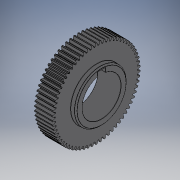
# Autodesk Inventor part: Component 16 (Sun Wheel)
Saved by Autodesk Inventor 2018 (Build 220112000, 112)
## iProperties
Created: 2023-03-15
Part Number: Component 16 (Sun Wheel)
Material: Generic
Document SubType Name: Modeling
Designer: Habib Mohamed
Density: 1 g/cm^3
Appearance: Semi-Polished
Author: Habib Mohamed
Autodesk Inventor part; units mm, degrees
(part 1 of 2)
ref_plane "YZ Plane" through (0, 0, 0) normal (1, 0, 0) x (0, 1, 0)
ref_plane "XZ Plane" through (0, 0, 0) normal (0, 1, 0) x (-1, 0, 0)
ref_plane "XY Plane" through (0, 0, 0) normal (0, 0, 1) x (1, 0, 0)
sketch "Sketch1" plane through (0, 0, 0) normal (1, 0, 0) x (0, 1, 0)
  line L0 (0, 0) -> (37.2988, 0) construction
  circle A0 centre (0, 0) radius 7.5
  line L1 (26.8131, 0.57) -> (11.4917, 0.57) construction
  line L2 (26.8131, 0.135) -> (10.3628, 0.135) construction
  arc A1 (16.9383, 0.2272) -> (15.9435, 0.5528) centre (14.4593, -5.6624) ccw
  arc A2 (16.9995, 0.135) -> (16.9383, 0.2272) centre (16.8995, 0.135) ccw
  arc A3 (15.8669, 0.646) -> (15.9435, 0.5528) centre (15.9668, 0.6501) ccw
  arc A4 (15.9435, -0.5528) -> (16.9383, -0.2272) centre (14.4593, 5.6624) ccw
  arc A5 (16.9383, -0.2272) -> (16.9995, -0.1358) centre (16.8995, -0.135) ccw
  arc A6 (15.9435, -0.5528) -> (15.8669, -0.646) centre (15.9668, -0.6501) ccw
  arc A7 (16.9097, 1.7503) -> (16.84, 1.8362) centre (16.8101, 1.7408) ccw
  arc A8 (15.7336, 2.1514) -> (15.8188, 2.0659) centre (15.8327, 2.1649) ccw
  arc A9 (16.8832, 1.3839) -> (16.9354, 1.4807) centre (16.8358, 1.472) ccw
  arc A10 (15.9239, 0.9652) -> (16.8832, 1.3839) centre (13.8556, 7.0112) ccw
  arc A11 (15.9239, 0.9652) -> (15.8564, 0.8651) centre (15.9563, 0.8706) ccw
  arc A12 (16.84, 1.8362) -> (15.8188, 2.0659) centre (14.9321, -4.2623) ccw
  arc A13 (16.6667, 3.3497) -> (16.5892, 3.4286) centre (16.5685, 3.3308) ccw
  arc A14 (15.4579, 3.6372) -> (15.5508, 3.5602) centre (15.5552, 3.6601) ccw
  arc A15 (16.6752, 2.9825) -> (16.718, 3.0838) centre (16.6196, 3.0657) ccw
  arc A16 (15.76, 2.4745) -> (16.6752, 2.9825) centre (13.1264, 8.2965) ccw
  arc A17 (15.76, 2.4745) -> (15.7024, 2.3685) centre (15.8013, 2.3834) ccw
  arc A18 (16.5892, 3.4286) -> (15.5508, 3.5602) centre (15.2696, -2.8236) ccw
  arc A19 (16.2728, 4.9188) -> (16.1881, 4.99) centre (16.1769, 4.8907) ccw
  arc A20 (15.0421, 5.0901) -> (15.142, 5.0223) centre (15.1368, 5.1221) ccw
  arc A21 (16.3161, 4.5541) -> (16.3491, 4.659) centre (16.2529, 4.6316) ccw
  arc A22 (15.4535, 3.9614) -> (16.3161, 4.5541) centre (12.2783, 9.5067) ccw
  arc A23 (15.4535, 3.9614) -> (15.4061, 3.8503) centre (15.5032, 3.8746) ccw
  arc A24 (16.1881, 4.99) -> (15.142, 5.0223) centre (15.4689, -1.3594) ccw
  arc A25 (15.7316, 6.4434) -> (15.6405, 6.5062) centre (15.6387, 6.4062) ccw
  arc A26 (14.4902, 6.4969) -> (14.596, 6.4389) centre (14.5814, 6.5378) ccw
  arc A27 (15.8094, 6.0844) -> (15.8322, 6.192) centre (15.7391, 6.1556) ccw
  arc A28 (15.0069, 5.4124) -> (15.8094, 6.0844) centre (11.3191, 10.6308) ccw
  arc A29 (15.0069, 5.4124) -> (14.9704, 5.2974) centre (15.0647, 5.3307) ccw
  arc A30 (15.6405, 6.5062) -> (14.596, 6.4389) centre (15.5281, 0.1172) ccw
  arc A31 (15.0479, 7.9096) -> (14.9512, 7.9635) centre (14.959, 7.8638) ccw
  arc A32 (13.807, 7.8448) -> (13.9179, 7.7971) centre (13.8939, 7.8942) ccw
  arc A33 (15.1594, 7.5596) -> (15.1719, 7.6689) centre (15.0827, 7.6238) ccw
  arc A34 (14.4245, 6.8144) -> (15.1594, 7.5596) centre (10.2573, 11.6586) ccw
  arc A35 (14.4245, 6.8144) -> (14.3991, 6.6964) centre (14.4897, 6.7386) ccw
  arc A36 (14.9512, 7.9635) -> (13.9179, 7.7971) centre (15.4466, 1.5927) ccw
  arc A37 (14.2279, 9.3042) -> (14.1266, 9.3486) centre (14.1437, 9.2501) ccw
  arc A38 (12.9988, 9.1218) -> (13.1137, 9.0848) centre (13.0806, 9.1792) ccw
  arc A39 (14.3722, 8.9664) -> (14.3743, 9.0764) centre (14.2897, 9.023) ccw
  arc A40 (13.7115, 8.1546) -> (14.3722, 8.9664) centre (9.1026, 12.5808) ccw
  arc A41 (13.7115, 8.1546) -> (13.6973, 8.0348) centre (13.7836, 8.0854) ccw
  arc A42 (14.1266, 9.3486) -> (13.1137, 9.0848) centre (15.2253, 3.0538) ccw
  arc A43 (13.279, 10.6145) -> (13.1739, 10.6491) centre (13.2004, 10.5527) ccw
  arc A44 (12.0728, 10.3161) -> (12.1907, 10.2902) centre (12.1489, 10.381) ccw
  arc A45 (13.4548, 10.292) -> (13.4464, 10.4016) centre (13.3673, 10.3404) ccw
  arc A46 (12.8742, 9.4211) -> (13.4548, 10.292) centre (7.8655, 13.3891) ccw
  arc A47 (12.8742, 9.4211) -> (12.8715, 9.3004) centre (12.9526, 9.359) ccw
  arc A48 (13.1739, 10.6491) -> (12.1907, 10.2902) centre (14.866, 4.4872) ccw
  arc A49 (12.2099, 11.8287) -> (12.102, 11.8531) centre (12.1376, 11.7597) ccw
  arc A50 (11.0376, 11.4169) -> (11.1574, 11.4024) centre (11.1071, 11.4888) ccw
  arc A51 (12.4156, 11.5243) -> (12.3968, 11.6327) centre (12.3239, 11.5643) ccw
  arc A52 (11.9204, 10.6022) -> (12.4156, 11.5243) centre (6.5572, 14.0761) ccw
  arc A53 (11.9204, 10.6022) -> (11.9292, 10.4818) centre (12.0043, 10.5478) ccw
  arc A54 (12.102, 11.8531) -> (11.1574, 11.4024) centre (14.3722, 5.88) ccw
  arc A55 (11.0303, 12.9357) -> (10.9205, 12.9498) centre (10.9648, 12.8602) ccw
  arc A56 (9.9023, 12.4144) -> (10.023, 12.4114) centre (9.9647, 12.4926) ccw
  arc A57 (11.2639, 12.6523) -> (11.2349, 12.7584) centre (11.1688, 12.6834) ccw
  arc A58 (10.8586, 11.6873) -> (11.2639, 12.6523) centre (5.1895, 14.6357) ccw
  arc A59 (10.8586, 11.6873) -> (10.8788, 11.5683) centre (10.9473, 11.6411) ccw
  arc A60 (10.9205, 12.9498) -> (10.023, 12.4114) centre (13.7482, 7.2195) ccw
  arc A61 (9.7507, 13.9257) -> (9.6401, 13.9293) centre (9.6927, 13.8442) ccw
  arc A62 (8.6774, 13.2995) -> (8.7978, 13.3079) centre (8.7321, 13.3832) ccw
  arc A63 (10.0102, 13.6657) -> (9.9713, 13.7686) centre (9.9126, 13.6876) ccw
  arc A64 (9.6985, 12.6665) -> (10.0102, 13.6657) centre (3.7748, 15.0627) ccw
  arc A65 (9.6985, 12.6665) -> (9.7299, 12.55) centre (9.7912, 12.629) ccw
  arc A66 (9.6401, 13.9293) -> (8.7978, 13.3079) centre (12.9997, 8.4937) ccw
  arc A67 (8.3828, 14.7895) -> (8.2724, 14.7825) centre (8.3328, 14.7029) ccw
  arc A68 (7.3739, 14.0641) -> (7.493, 14.0839) centre (7.4204, 14.1527) ccw
  arc A69 (8.6659, 14.5554) -> (8.6173, 14.6541) centre (8.5666, 14.5679) ccw
  arc A70 (8.4505, 13.5311) -> (8.6659, 14.5554) centre (2.3259, 15.3533) ccw
  arc A71 (8.4505, 13.5311) -> (8.4929, 13.4181) centre (8.5464, 13.5026) ccw
  arc A72 (8.2724, 14.7825) -> (7.493, 14.0839) centre (12.1334, 9.6909) ccw
  arc A73 (6.939, 15.5193) -> (6.8298, 15.5019) centre (6.8975, 15.4284) ccw
  arc A74 (6.0037, 14.7014) -> (6.1203, 14.7324) centre (6.0415, 14.794) ccw
  arc A75 (7.243, 15.3132) -> (7.1854, 15.4068) centre (7.1431, 15.3162) ccw
  arc A76 (7.1261, 14.2731) -> (7.243, 15.3132) centre (0.8559, 15.5049) ccw
  arc A77 (7.1261, 14.2731) -> (7.179, 14.1646) centre (7.2242, 14.2538) ccw
  arc A78 (6.8298, 15.5019) -> (6.1203, 14.7324) centre (11.1573, 10.8004) ccw
  arc A79 (5.4324, 16.1087) -> (5.3253, 16.081) centre (5.3997, 16.0142) ccw
  arc A80 (4.579, 15.2055) -> (4.6922, 15.2475) centre (4.6079, 15.3012) ccw
  arc A81 (5.7546, 15.9324) -> (5.6883, 16.0201) centre (5.6548, 15.9259) ccw
  arc A82 (5.7371, 14.8858) -> (5.7546, 15.9324) centre (-0.6218, 15.516) ccw
  arc A83 (5.7371, 14.8858) -> (5.8, 14.7829) centre (5.8366, 14.876) ccw
  arc A84 (5.3253, 16.081) -> (4.6922, 15.2475) centre (10.0801, 11.8121) ccw
  arc A85 (3.8766, 16.5521) -> (3.7726, 16.5143) centre (3.853, 16.4549) ccw
  arc A86 (3.1129, 15.5719) -> (3.2216, 15.6245) centre (3.1325, 15.67) ccw
  arc A87 (4.2141, 16.4072) -> (4.1397, 16.4883) centre (4.1154, 16.3913) ccw
  arc A88 (4.2961, 15.3638) -> (4.2141, 16.4072) centre (-2.0939, 15.3867) ccw
  arc A89 (4.2961, 15.3638) -> (4.3686, 15.2673) centre (4.3961, 15.3634) ccw
  arc A90 (3.7726, 16.5143) -> (3.2216, 15.6245) centre (8.9117, 12.7168) ccw
  arc A91 (2.2856, 16.8456) -> (2.1857, 16.7982) centre (2.2714, 16.7467) ccw
  arc A92 (1.6186, 15.7973) -> (1.7218, 15.8599) centre (1.6288, 15.8968) ccw
  arc A93 (2.6354, 16.7335) -> (2.5537, 16.8071) centre (2.5387, 16.7082) ccw
  arc A94 (2.8162, 15.7026) -> (2.6354, 16.7335) centre (-3.547, 15.118) ccw
  arc A95 (2.8162, 15.7026) -> (2.8976, 15.6134) centre (2.9158, 15.7117) ccw
  arc A96 (2.1857, 16.7982) -> (1.7218, 15.8599) centre (7.6625, 13.5063) ccw
  arc A97 (0.674, 16.9866) -> (0.579, 16.9299) centre (0.6693, 16.8867) ccw
  arc A98 (0.1097, 15.8796) -> (0.2064, 15.9518) centre (0.1104, 15.9796) ccw
  arc A99 (1.0329, 16.9083) -> (0.9445, 16.9737) centre (0.939, 16.8739) ccw
  arc A100 (1.3108, 15.8992) -> (1.0329, 16.9083) centre (-4.968, 14.7124) ccw
  arc A101 (1.3108, 15.8992) -> (1.4003, 15.8181) centre (1.4091, 15.9178) ccw
  arc A102 (0.579, 16.9299) -> (0.2064, 15.9518) centre (6.344, 14.1735) ccw
  arc A103 (-0.9437, 16.9738) -> (-1.0329, 16.9083) centre (-0.939, 16.8739) ccw
  arc A104 (-1.4003, 15.8181) -> (-1.3108, 15.8992) centre (-1.4091, 15.9178) ccw
  arc A105 (-0.579, 16.9299) -> (-0.6732, 16.9867) centre (-0.6693, 16.8867) ccw
  arc A106 (-0.2064, 15.9518) -> (-0.579, 16.9299) centre (-6.344, 14.1735) ccw
  arc A107 (-0.2064, 15.9518) -> (-0.1097, 15.8796) centre (-0.1104, 15.9796) ccw
  arc A108 (-1.0329, 16.9083) -> (-1.3108, 15.8992) centre (4.968, 14.7124) ccw
  arc A109 (-2.5529, 16.8072) -> (-2.6354, 16.7335) centre (-2.5387, 16.7082) ccw
  arc A110 (-2.8976, 15.6134) -> (-2.8162, 15.7026) centre (-2.9158, 15.7117) ccw
  arc A111 (-2.1857, 16.7982) -> (-2.2849, 16.8458) centre (-2.2714, 16.7467) ccw
  arc A112 (-1.7218, 15.8599) -> (-2.1857, 16.7982) centre (-7.6625, 13.5063) ccw
  arc A113 (-1.7218, 15.8599) -> (-1.6186, 15.7973) centre (-1.6288, 15.8968) ccw
  arc A114 (-2.6354, 16.7335) -> (-2.8162, 15.7026) centre (3.547, 15.118) ccw
  arc A115 (-4.139, 16.4884) -> (-4.2141, 16.4072) centre (-4.1154, 16.3913) ccw
  arc A116 (-4.3686, 15.2673) -> (-4.2961, 15.3638) centre (-4.3961, 15.3634) ccw
  arc A117 (-3.7726, 16.5143) -> (-3.8758, 16.5523) centre (-3.853, 16.4549) ccw
  arc A118 (-3.2216, 15.6245) -> (-3.7726, 16.5143) centre (-8.9117, 12.7168) ccw
  arc A119 (-3.2216, 15.6245) -> (-3.1129, 15.5719) centre (-3.1325, 15.67) ccw
  arc A120 (-4.2141, 16.4072) -> (-4.2961, 15.3638) centre (2.0939, 15.3867) ccw
  arc A121 (-5.6876, 16.0204) -> (-5.7546, 15.9324) centre (-5.6548, 15.9259) ccw
  arc A122 (-5.8, 14.7829) -> (-5.7371, 14.8858) centre (-5.8366, 14.876) ccw
  arc A123 (-5.3253, 16.081) -> (-5.4316, 16.1089) centre (-5.3997, 16.0142) ccw
  arc A124 (-4.6922, 15.2475) -> (-5.3253, 16.081) centre (-10.0801, 11.8121) ccw
  arc A125 (-4.6922, 15.2475) -> (-4.579, 15.2055) centre (-4.6079, 15.3012) ccw
  arc A126 (-5.7546, 15.9324) -> (-5.7371, 14.8858) centre (0.6218, 15.516) ccw
  arc A127 (-7.1846, 15.4072) -> (-7.243, 15.3132) centre (-7.1431, 15.3162) ccw
  arc A128 (-7.179, 14.1646) -> (-7.1261, 14.2731) centre (-7.2242, 14.2538) ccw
  arc A129 (-6.8298, 15.5019) -> (-6.9383, 15.5197) centre (-6.8975, 15.4284) ccw
  arc A130 (-6.1203, 14.7324) -> (-6.8298, 15.5019) centre (-11.1573, 10.8004) ccw
  arc A131 (-6.1203, 14.7324) -> (-6.0037, 14.7014) centre (-6.0415, 14.794) ccw
  arc A132 (-7.243, 15.3132) -> (-7.1261, 14.2731) centre (-0.8559, 15.5049) ccw
  arc A133 (-8.6166, 14.6545) -> (-8.6659, 14.5554) centre (-8.5666, 14.5679) ccw
  arc A134 (-8.4929, 13.4181) -> (-8.4505, 13.5311) centre (-8.5464, 13.5026) ccw
  arc A135 (-8.2724, 14.7825) -> (-8.3821, 14.7899) centre (-8.3328, 14.7029) ccw
  arc A136 (-7.493, 14.0839) -> (-8.2724, 14.7825) centre (-12.1334, 9.6909) ccw
  arc A137 (-7.493, 14.0839) -> (-7.3739, 14.0641) centre (-7.4204, 14.1527) ccw
  arc A138 (-8.6659, 14.5554) -> (-8.4505, 13.5311) centre (-2.3259, 15.3533) ccw
  arc A139 (-9.9706, 13.769) -> (-10.0102, 13.6657) centre (-9.9126, 13.6876) ccw
  arc A140 (-9.7299, 12.55) -> (-9.6985, 12.6665) centre (-9.7912, 12.629) ccw
  arc A141 (-9.6401, 13.9293) -> (-9.75, 13.9261) centre (-9.6927, 13.8442) ccw
  arc A142 (-8.7978, 13.3079) -> (-9.6401, 13.9293) centre (-12.9997, 8.4937) ccw
  arc A143 (-8.7978, 13.3079) -> (-8.6774, 13.2995) centre (-8.7321, 13.3832) ccw
  arc A144 (-10.0102, 13.6657) -> (-9.6985, 12.6665) centre (-3.7748, 15.0627) ccw
  arc A145 (-11.2343, 12.7589) -> (-11.2639, 12.6523) centre (-11.1688, 12.6834) ccw
  arc A146 (-10.8788, 11.5683) -> (-10.8586, 11.6873) centre (-10.9473, 11.6411) ccw
  arc A147 (-10.9205, 12.9498) -> (-11.0296, 12.9363) centre (-10.9648, 12.8602) ccw
  arc A148 (-10.023, 12.4114) -> (-10.9205, 12.9498) centre (-13.7482, 7.2195) ccw
  arc A149 (-10.023, 12.4114) -> (-9.9023, 12.4144) centre (-9.9647, 12.4926) ccw
  arc A150 (-11.2639, 12.6523) -> (-10.8586, 11.6873) centre (-5.1895, 14.6357) ccw
  arc A151 (-12.3962, 11.6333) -> (-12.4156, 11.5243) centre (-12.3239, 11.5643) ccw
  arc A152 (-11.9292, 10.4818) -> (-11.9204, 10.6022) centre (-12.0043, 10.5478) ccw
  arc A153 (-12.102, 11.8531) -> (-12.2094, 11.8293) centre (-12.1376, 11.7597) ccw
  arc A154 (-11.1574, 11.4024) -> (-12.102, 11.8531) centre (-14.3722, 5.88) ccw
  arc A155 (-11.1574, 11.4024) -> (-11.0376, 11.4169) centre (-11.1071, 11.4888) ccw
  arc A156 (-12.4156, 11.5243) -> (-11.9204, 10.6022) centre (-6.5572, 14.0761) ccw
  arc A157 (-13.4459, 10.4023) -> (-13.4548, 10.292) centre (-13.3673, 10.3404) ccw
  arc A158 (-12.8715, 9.3004) -> (-12.8742, 9.4211) centre (-12.9526, 9.359) ccw
  arc A159 (-13.1739, 10.6491) -> (-13.2785, 10.6151) centre (-13.2004, 10.5527) ccw
  arc A160 (-12.1907, 10.2902) -> (-13.1739, 10.6491) centre (-14.866, 4.4872) ccw
  arc A161 (-12.1907, 10.2902) -> (-12.0728, 10.3161) centre (-12.1489, 10.381) ccw
  arc A162 (-13.4548, 10.292) -> (-12.8742, 9.4211) centre (-7.8655, 13.3891) ccw
  arc A163 (-14.3738, 9.077) -> (-14.3722, 8.9664) centre (-14.2897, 9.023) ccw
  arc A164 (-13.6973, 8.0348) -> (-13.7115, 8.1546) centre (-13.7836, 8.0854) ccw
  arc A165 (-14.1266, 9.3486) -> (-14.2274, 9.3048) centre (-14.1437, 9.2501) ccw
  arc A166 (-13.1137, 9.0848) -> (-14.1266, 9.3486) centre (-15.2253, 3.0538) ccw
  arc A167 (-13.1137, 9.0848) -> (-12.9988, 9.1218) centre (-13.0806, 9.1792) ccw
  arc A168 (-14.3722, 8.9664) -> (-13.7115, 8.1546) centre (-9.1026, 12.5808) ccw
  arc A169 (-15.1716, 7.6696) -> (-15.1594, 7.5596) centre (-15.0827, 7.6238) ccw
  arc A170 (-14.3991, 6.6964) -> (-14.4245, 6.8144) centre (-14.4897, 6.7386) ccw
  arc A171 (-14.9512, 7.9635) -> (-15.0475, 7.9103) centre (-14.959, 7.8638) ccw
  arc A172 (-13.9179, 7.7971) -> (-14.9512, 7.9635) centre (-15.4466, 1.5927) ccw
  arc A173 (-13.9179, 7.7971) -> (-13.807, 7.8448) centre (-13.8939, 7.8942) ccw
  arc A174 (-15.1594, 7.5596) -> (-14.4245, 6.8144) centre (-10.2573, 11.6586) ccw
  arc A175 (-15.8319, 6.1927) -> (-15.8094, 6.0844) centre (-15.7391, 6.1556) ccw
  arc A176 (-14.9704, 5.2974) -> (-15.0069, 5.4124) centre (-15.0647, 5.3307) ccw
  arc A177 (-15.6405, 6.5062) -> (-15.7313, 6.4441) centre (-15.6387, 6.4062) ccw
  arc A178 (-14.596, 6.4389) -> (-15.6405, 6.5062) centre (-15.5281, 0.1172) ccw
  arc A179 (-14.596, 6.4389) -> (-14.4902, 6.4969) centre (-14.5814, 6.5378) ccw
  arc A180 (-15.8094, 6.0844) -> (-15.0069, 5.4124) centre (-11.3191, 10.6308) ccw
  arc A181 (-16.3489, 4.6598) -> (-16.3161, 4.5541) centre (-16.2529, 4.6316) ccw
  arc A182 (-15.4061, 3.8503) -> (-15.4535, 3.9614) centre (-15.5032, 3.8746) ccw
  arc A183 (-16.1881, 4.99) -> (-16.2726, 4.9196) centre (-16.1769, 4.8907) ccw
  arc A184 (-15.142, 5.0223) -> (-16.1881, 4.99) centre (-15.4689, -1.3594) ccw
  arc A185 (-15.142, 5.0223) -> (-15.0421, 5.0901) centre (-15.1368, 5.1221) ccw
  arc A186 (-16.3161, 4.5541) -> (-15.4535, 3.9614) centre (-12.2783, 9.5067) ccw
  arc A187 (-16.7178, 3.0846) -> (-16.6752, 2.9825) centre (-16.6196, 3.0657) ccw
  arc A188 (-15.7024, 2.3685) -> (-15.76, 2.4745) centre (-15.8013, 2.3834) ccw
  arc A189 (-16.5892, 3.4286) -> (-16.6666, 3.3505) centre (-16.5685, 3.3308) ccw
  arc A190 (-15.5508, 3.5602) -> (-16.5892, 3.4286) centre (-15.2696, -2.8236) ccw
  arc A191 (-15.5508, 3.5602) -> (-15.4579, 3.6372) centre (-15.5552, 3.6601) ccw
  arc A192 (-16.6752, 2.9825) -> (-15.76, 2.4745) centre (-13.1264, 8.2965) ccw
  arc A193 (-16.9353, 1.4815) -> (-16.8832, 1.3839) centre (-16.8358, 1.472) ccw
  arc A194 (-15.8564, 0.8651) -> (-15.9239, 0.9652) centre (-15.9563, 0.8706) ccw
  arc A195 (-16.84, 1.8362) -> (-16.9096, 1.7511) centre (-16.8101, 1.7408) ccw
  arc A196 (-15.8188, 2.0659) -> (-16.84, 1.8362) centre (-14.9321, -4.2623) ccw
  arc A197 (-15.8188, 2.0659) -> (-15.7336, 2.1514) centre (-15.8327, 2.1649) ccw
  arc A198 (-16.8832, 1.3839) -> (-15.9239, 0.9652) centre (-13.8556, 7.0112) ccw
  arc A199 (-16.9995, -0.135) -> (-16.9383, -0.2272) centre (-16.8995, -0.135) ccw
  arc A200 (-15.8669, -0.646) -> (-15.9435, -0.5528) centre (-15.9668, -0.6501) ccw
  arc A201 (-16.9383, 0.2272) -> (-16.9995, 0.1358) centre (-16.8995, 0.135) ccw
  arc A202 (-15.9435, 0.5528) -> (-16.9383, 0.2272) centre (-14.4593, -5.6624) ccw
  arc A203 (-15.9435, 0.5528) -> (-15.8669, 0.646) centre (-15.9668, 0.6501) ccw
  arc A204 (-16.9383, -0.2272) -> (-15.9435, -0.5528) centre (-14.4593, 5.6624) ccw
  arc A205 (-16.9097, -1.7503) -> (-16.84, -1.8362) centre (-16.8101, -1.7408) ccw
  arc A206 (-15.7336, -2.1514) -> (-15.8188, -2.0659) centre (-15.8327, -2.1649) ccw
  arc A207 (-16.8832, -1.3839) -> (-16.9354, -1.4807) centre (-16.8358, -1.472) ccw
  arc A208 (-15.9239, -0.9652) -> (-16.8832, -1.3839) centre (-13.8556, -7.0112) ccw
  arc A209 (-15.9239, -0.9652) -> (-15.8564, -0.8651) centre (-15.9563, -0.8706) ccw
  arc A210 (-16.84, -1.8362) -> (-15.8188, -2.0659) centre (-14.9321, 4.2623) ccw
  arc A211 (-16.6667, -3.3497) -> (-16.5892, -3.4286) centre (-16.5685, -3.3308) ccw
  arc A212 (-15.4579, -3.6372) -> (-15.5508, -3.5602) centre (-15.5552, -3.6601) ccw
  arc A213 (-16.6752, -2.9825) -> (-16.718, -3.0838) centre (-16.6196, -3.0657) ccw
  arc A214 (-15.76, -2.4745) -> (-16.6752, -2.9825) centre (-13.1264, -8.2965) ccw
  arc A215 (-15.76, -2.4745) -> (-15.7024, -2.3685) centre (-15.8013, -2.3834) ccw
  arc A216 (-16.5892, -3.4286) -> (-15.5508, -3.5602) centre (-15.2696, 2.8236) ccw
  arc A217 (-16.2728, -4.9188) -> (-16.1881, -4.99) centre (-16.1769, -4.8907) ccw
  arc A218 (-15.0421, -5.0901) -> (-15.142, -5.0223) centre (-15.1368, -5.1221) ccw
  arc A219 (-16.3161, -4.5541) -> (-16.3491, -4.659) centre (-16.2529, -4.6316) ccw
  arc A220 (-15.4535, -3.9614) -> (-16.3161, -4.5541) centre (-12.2783, -9.5067) ccw
  arc A221 (-15.4535, -3.9614) -> (-15.4061, -3.8503) centre (-15.5032, -3.8746) ccw
  arc A222 (-16.1881, -4.99) -> (-15.142, -5.0223) centre (-15.4689, 1.3594) ccw
  arc A223 (-15.7316, -6.4434) -> (-15.6405, -6.5062) centre (-15.6387, -6.4062) ccw
  arc A224 (-14.4902, -6.4969) -> (-14.596, -6.4389) centre (-14.5814, -6.5378) ccw
  arc A225 (-15.8094, -6.0844) -> (-15.8322, -6.192) centre (-15.7391, -6.1556) ccw
  arc A226 (-15.0069, -5.4124) -> (-15.8094, -6.0844) centre (-11.3191, -10.6308) ccw
  arc A227 (-15.0069, -5.4124) -> (-14.9704, -5.2974) centre (-15.0647, -5.3307) ccw
  arc A228 (-15.6405, -6.5062) -> (-14.596, -6.4389) centre (-15.5281, -0.1172) ccw
  arc A229 (-15.0479, -7.9096) -> (-14.9512, -7.9635) centre (-14.959, -7.8638) ccw
  arc A230 (-13.807, -7.8448) -> (-13.9179, -7.7971) centre (-13.8939, -7.8942) ccw
  arc A231 (-15.1594, -7.5596) -> (-15.1719, -7.6689) centre (-15.0827, -7.6238) ccw
  arc A232 (-14.4245, -6.8144) -> (-15.1594, -7.5596) centre (-10.2573, -11.6586) ccw
  arc A233 (-14.4245, -6.8144) -> (-14.3991, -6.6964) centre (-14.4897, -6.7386) ccw
  arc A234 (-14.9512, -7.9635) -> (-13.9179, -7.7971) centre (-15.4466, -1.5927) ccw
  arc A235 (-14.2279, -9.3042) -> (-14.1266, -9.3486) centre (-14.1437, -9.2501) ccw
  arc A236 (-12.9988, -9.1218) -> (-13.1137, -9.0848) centre (-13.0806, -9.1792) ccw
  arc A237 (-14.3722, -8.9664) -> (-14.3743, -9.0764) centre (-14.2897, -9.023) ccw
  arc A238 (-13.7115, -8.1546) -> (-14.3722, -8.9664) centre (-9.1026, -12.5808) ccw
  arc A239 (-13.7115, -8.1546) -> (-13.6973, -8.0348) centre (-13.7836, -8.0854) ccw
  arc A240 (-14.1266, -9.3486) -> (-13.1137, -9.0848) centre (-15.2253, -3.0538) ccw
  arc A241 (-13.279, -10.6145) -> (-13.1739, -10.6491) centre (-13.2004, -10.5527) ccw
  arc A242 (-12.0728, -10.3161) -> (-12.1907, -10.2902) centre (-12.1489, -10.381) ccw
  arc A243 (-13.4548, -10.292) -> (-13.4464, -10.4016) centre (-13.3673, -10.3404) ccw
  arc A244 (-12.8742, -9.4211) -> (-13.4548, -10.292) centre (-7.8655, -13.3891) ccw
  arc A245 (-12.8742, -9.4211) -> (-12.8715, -9.3004) centre (-12.9526, -9.359) ccw
  arc A246 (-13.1739, -10.6491) -> (-12.1907, -10.2902) centre (-14.866, -4.4872) ccw
  arc A247 (-12.2099, -11.8287) -> (-12.102, -11.8531) centre (-12.1376, -11.7597) ccw
  arc A248 (-11.0376, -11.4169) -> (-11.1574, -11.4024) centre (-11.1071, -11.4888) ccw
  arc A249 (-12.4156, -11.5243) -> (-12.3968, -11.6327) centre (-12.3239, -11.5643) ccw
  arc A250 (-11.9204, -10.6022) -> (-12.4156, -11.5243) centre (-6.5572, -14.0761) ccw
  arc A251 (-11.9204, -10.6022) -> (-11.9292, -10.4818) centre (-12.0043, -10.5478) ccw
  arc A252 (-12.102, -11.8531) -> (-11.1574, -11.4024) centre (-14.3722, -5.88) ccw
  arc A253 (-11.0303, -12.9357) -> (-10.9205, -12.9498) centre (-10.9648, -12.8602) ccw
  arc A254 (-9.9023, -12.4144) -> (-10.023, -12.4114) centre (-9.9647, -12.4926) ccw
  arc A255 (-11.2639, -12.6523) -> (-11.2349, -12.7584) centre (-11.1688, -12.6834) ccw
  arc A256 (-10.8586, -11.6873) -> (-11.2639, -12.6523) centre (-5.1895, -14.6357) ccw
  arc A257 (-10.8586, -11.6873) -> (-10.8788, -11.5683) centre (-10.9473, -11.6411) ccw
  arc A258 (-10.9205, -12.9498) -> (-10.023, -12.4114) centre (-13.7482, -7.2195) ccw
  arc A259 (-9.7507, -13.9257) -> (-9.6401, -13.9293) centre (-9.6927, -13.8442) ccw
  arc A260 (-8.6774, -13.2995) -> (-8.7978, -13.3079) centre (-8.7321, -13.3832) ccw
  arc A261 (-10.0102, -13.6657) -> (-9.9713, -13.7686) centre (-9.9126, -13.6876) ccw
  arc A262 (-9.6985, -12.6665) -> (-10.0102, -13.6657) centre (-3.7748, -15.0627) ccw
  arc A263 (-9.6985, -12.6665) -> (-9.7299, -12.55) centre (-9.7912, -12.629) ccw
  arc A264 (-9.6401, -13.9293) -> (-8.7978, -13.3079) centre (-12.9997, -8.4937) ccw
  arc A265 (-8.3828, -14.7895) -> (-8.2724, -14.7825) centre (-8.3328, -14.7029) ccw
  arc A266 (-7.3739, -14.0641) -> (-7.493, -14.0839) centre (-7.4204, -14.1527) ccw
  arc A267 (-8.6659, -14.5554) -> (-8.6173, -14.6541) centre (-8.5666, -14.5679) ccw
  arc A268 (-8.4505, -13.5311) -> (-8.6659, -14.5554) centre (-2.3259, -15.3533) ccw
  arc A269 (-8.4505, -13.5311) -> (-8.4929, -13.4181) centre (-8.5464, -13.5026) ccw
  arc A270 (-8.2724, -14.7825) -> (-7.493, -14.0839) centre (-12.1334, -9.6909) ccw
  arc A271 (-6.939, -15.5193) -> (-6.8298, -15.5019) centre (-6.8975, -15.4284) ccw
  arc A272 (-6.0037, -14.7014) -> (-6.1203, -14.7324) centre (-6.0415, -14.794) ccw
  arc A273 (-7.243, -15.3132) -> (-7.1854, -15.4068) centre (-7.1431, -15.3162) ccw
  arc A274 (-7.1261, -14.2731) -> (-7.243, -15.3132) centre (-0.8559, -15.5049) ccw
  arc A275 (-7.1261, -14.2731) -> (-7.179, -14.1646) centre (-7.2242, -14.2538) ccw
  arc A276 (-6.8298, -15.5019) -> (-6.1203, -14.7324) centre (-11.1573, -10.8004) ccw
  arc A277 (-5.4324, -16.1087) -> (-5.3253, -16.081) centre (-5.3997, -16.0142) ccw
  arc A278 (-4.579, -15.2055) -> (-4.6922, -15.2475) centre (-4.6079, -15.3012) ccw
  arc A279 (-5.7546, -15.9324) -> (-5.6883, -16.0201) centre (-5.6548, -15.9259) ccw
  arc A280 (-5.7371, -14.8858) -> (-5.7546, -15.9324) centre (0.6218, -15.516) ccw
  arc A281 (-5.7371, -14.8858) -> (-5.8, -14.7829) centre (-5.8366, -14.876) ccw
  arc A282 (-5.3253, -16.081) -> (-4.6922, -15.2475) centre (-10.0801, -11.8121) ccw
  arc A283 (-3.8766, -16.5521) -> (-3.7726, -16.5143) centre (-3.853, -16.4549) ccw
  arc A284 (-3.1129, -15.5719) -> (-3.2216, -15.6245) centre (-3.1325, -15.67) ccw
  arc A285 (-4.2141, -16.4072) -> (-4.1397, -16.4883) centre (-4.1154, -16.3913) ccw
  arc A286 (-4.2961, -15.3638) -> (-4.2141, -16.4072) centre (2.0939, -15.3867) ccw
  arc A287 (-4.2961, -15.3638) -> (-4.3686, -15.2673) centre (-4.3961, -15.3634) ccw
  arc A288 (-3.7726, -16.5143) -> (-3.2216, -15.6245) centre (-8.9117, -12.7168) ccw
  arc A289 (-2.2856, -16.8456) -> (-2.1857, -16.7982) centre (-2.2714, -16.7467) ccw
  arc A290 (-1.6186, -15.7973) -> (-1.7218, -15.8599) centre (-1.6288, -15.8968) ccw
  arc A291 (-2.6354, -16.7335) -> (-2.5537, -16.8071) centre (-2.5387, -16.7082) ccw
  arc A292 (-2.8162, -15.7026) -> (-2.6354, -16.7335) centre (3.547, -15.118) ccw
  arc A293 (-2.8162, -15.7026) -> (-2.8976, -15.6134) centre (-2.9158, -15.7117) ccw
  arc A294 (-2.1857, -16.7982) -> (-1.7218, -15.8599) centre (-7.6625, -13.5063) ccw
  arc A295 (-0.674, -16.9866) -> (-0.579, -16.9299) centre (-0.6693, -16.8867) ccw
  arc A296 (-0.1097, -15.8796) -> (-0.2064, -15.9518) centre (-0.1104, -15.9796) ccw
  arc A297 (-1.0329, -16.9083) -> (-0.9445, -16.9737) centre (-0.939, -16.8739) ccw
  arc A298 (-1.3108, -15.8992) -> (-1.0329, -16.9083) centre (4.968, -14.7124) ccw
  arc A299 (-1.3108, -15.8992) -> (-1.4003, -15.8181) centre (-1.4091, -15.9178) ccw
  arc A300 (-0.579, -16.9299) -> (-0.2064, -15.9518) centre (-6.344, -14.1735) ccw
  arc A301 (0.9437, -16.9738) -> (1.0329, -16.9083) centre (0.939, -16.8739) ccw
  arc A302 (1.4003, -15.8181) -> (1.3108, -15.8992) centre (1.4091, -15.9178) ccw
  arc A303 (0.579, -16.9299) -> (0.6732, -16.9867) centre (0.6693, -16.8867) ccw
  arc A304 (0.2064, -15.9518) -> (0.579, -16.9299) centre (6.344, -14.1735) ccw
  arc A305 (0.2064, -15.9518) -> (0.1097, -15.8796) centre (0.1104, -15.9796) ccw
  arc A306 (1.0329, -16.9083) -> (1.3108, -15.8992) centre (-4.968, -14.7124) ccw
  arc A307 (2.5529, -16.8072) -> (2.6354, -16.7335) centre (2.5387, -16.7082) ccw
  arc A308 (2.8976, -15.6134) -> (2.8162, -15.7026) centre (2.9158, -15.7117) ccw
  arc A309 (2.1857, -16.7982) -> (2.2849, -16.8458) centre (2.2714, -16.7467) ccw
  arc A310 (1.7218, -15.8599) -> (2.1857, -16.7982) centre (7.6625, -13.5063) ccw
  arc A311 (1.7218, -15.8599) -> (1.6186, -15.7973) centre (1.6288, -15.8968) ccw
  arc A312 (2.6354, -16.7335) -> (2.8162, -15.7026) centre (-3.547, -15.118) ccw
  arc A313 (4.139, -16.4884) -> (4.2141, -16.4072) centre (4.1154, -16.3913) ccw
  arc A314 (4.3686, -15.2673) -> (4.2961, -15.3638) centre (4.3961, -15.3634) ccw
  arc A315 (3.7726, -16.5143) -> (3.8758, -16.5523) centre (3.853, -16.4549) ccw
  arc A316 (3.2216, -15.6245) -> (3.7726, -16.5143) centre (8.9117, -12.7168) ccw
  arc A317 (3.2216, -15.6245) -> (3.1129, -15.5719) centre (3.1325, -15.67) ccw
  arc A318 (4.2141, -16.4072) -> (4.2961, -15.3638) centre (-2.0939, -15.3867) ccw
  arc A319 (5.6876, -16.0204) -> (5.7546, -15.9324) centre (5.6548, -15.9259) ccw
  arc A320 (5.8, -14.7829) -> (5.7371, -14.8858) centre (5.8366, -14.876) ccw
  arc A321 (5.3253, -16.081) -> (5.4316, -16.1089) centre (5.3997, -16.0142) ccw
  arc A322 (4.6922, -15.2475) -> (5.3253, -16.081) centre (10.0801, -11.8121) ccw
  arc A323 (4.6922, -15.2475) -> (4.579, -15.2055) centre (4.6079, -15.3012) ccw
  arc A324 (5.7546, -15.9324) -> (5.7371, -14.8858) centre (-0.6218, -15.516) ccw
  arc A325 (7.1846, -15.4072) -> (7.243, -15.3132) centre (7.1431, -15.3162) ccw
  arc A326 (7.179, -14.1646) -> (7.1261, -14.2731) centre (7.2242, -14.2538) ccw
  arc A327 (6.8298, -15.5019) -> (6.9383, -15.5197) centre (6.8975, -15.4284) ccw
  arc A328 (6.1203, -14.7324) -> (6.8298, -15.5019) centre (11.1573, -10.8004) ccw
  arc A329 (6.1203, -14.7324) -> (6.0037, -14.7014) centre (6.0415, -14.794) ccw
  arc A330 (7.243, -15.3132) -> (7.1261, -14.2731) centre (0.8559, -15.5049) ccw
  arc A331 (8.6166, -14.6545) -> (8.6659, -14.5554) centre (8.5666, -14.5679) ccw
  arc A332 (8.4929, -13.4181) -> (8.4505, -13.5311) centre (8.5464, -13.5026) ccw
  arc A333 (8.2724, -14.7825) -> (8.3821, -14.7899) centre (8.3328, -14.7029) ccw
  arc A334 (7.493, -14.0839) -> (8.2724, -14.7825) centre (12.1334, -9.6909) ccw
  arc A335 (7.493, -14.0839) -> (7.3739, -14.0641) centre (7.4204, -14.1527) ccw
  arc A336 (8.6659, -14.5554) -> (8.4505, -13.5311) centre (2.3259, -15.3533) ccw
  arc A337 (9.9706, -13.769) -> (10.0102, -13.6657) centre (9.9126, -13.6876) ccw
  arc A338 (9.7299, -12.55) -> (9.6985, -12.6665) centre (9.7912, -12.629) ccw
  arc A339 (9.6401, -13.9293) -> (9.75, -13.9261) centre (9.6927, -13.8442) ccw
  arc A340 (8.7978, -13.3079) -> (9.6401, -13.9293) centre (12.9997, -8.4937) ccw
  arc A341 (8.7978, -13.3079) -> (8.6774, -13.2995) centre (8.7321, -13.3832) ccw
  arc A342 (10.0102, -13.6657) -> (9.6985, -12.6665) centre (3.7748, -15.0627) ccw
  arc A343 (11.2343, -12.7589) -> (11.2639, -12.6523) centre (11.1688, -12.6834) ccw
  arc A344 (10.8788, -11.5683) -> (10.8586, -11.6873) centre (10.9473, -11.6411) ccw
  arc A345 (10.9205, -12.9498) -> (11.0296, -12.9363) centre (10.9648, -12.8602) ccw
  arc A346 (10.023, -12.4114) -> (10.9205, -12.9498) centre (13.7482, -7.2195) ccw
  arc A347 (10.023, -12.4114) -> (9.9023, -12.4144) centre (9.9647, -12.4926) ccw
  arc A348 (11.2639, -12.6523) -> (10.8586, -11.6873) centre (5.1895, -14.6357) ccw
  arc A349 (12.3962, -11.6333) -> (12.4156, -11.5243) centre (12.3239, -11.5643) ccw
  arc A350 (11.9292, -10.4818) -> (11.9204, -10.6022) centre (12.0043, -10.5478) ccw
  arc A351 (12.102, -11.8531) -> (12.2094, -11.8293) centre (12.1376, -11.7597) ccw
  arc A352 (11.1574, -11.4024) -> (12.102, -11.8531) centre (14.3722, -5.88) ccw
  arc A353 (11.1574, -11.4024) -> (11.0376, -11.4169) centre (11.1071, -11.4888) ccw
  arc A354 (12.4156, -11.5243) -> (11.9204, -10.6022) centre (6.5572, -14.0761) ccw
  arc A355 (13.4459, -10.4023) -> (13.4548, -10.292) centre (13.3673, -10.3404) ccw
  arc A356 (12.8715, -9.3004) -> (12.8742, -9.4211) centre (12.9526, -9.359) ccw
  arc A357 (13.1739, -10.6491) -> (13.2785, -10.6151) centre (13.2004, -10.5527) ccw
  arc A358 (12.1907, -10.2902) -> (13.1739, -10.6491) centre (14.866, -4.4872) ccw
  arc A359 (12.1907, -10.2902) -> (12.0728, -10.3161) centre (12.1489, -10.381) ccw
  arc A360 (13.4548, -10.292) -> (12.8742, -9.4211) centre (7.8655, -13.3891) ccw
  arc A361 (14.3738, -9.077) -> (14.3722, -8.9664) centre (14.2897, -9.023) ccw
  arc A362 (13.6973, -8.0348) -> (13.7115, -8.1546) centre (13.7836, -8.0854) ccw
  arc A363 (14.1266, -9.3486) -> (14.2274, -9.3048) centre (14.1437, -9.2501) ccw
  arc A364 (13.1137, -9.0848) -> (14.1266, -9.3486) centre (15.2253, -3.0538) ccw
  arc A365 (13.1137, -9.0848) -> (12.9988, -9.1218) centre (13.0806, -9.1792) ccw
  arc A366 (14.3722, -8.9664) -> (13.7115, -8.1546) centre (9.1026, -12.5808) ccw
  arc A367 (15.1716, -7.6696) -> (15.1594, -7.5596) centre (15.0827, -7.6238) ccw
  arc A368 (14.3991, -6.6964) -> (14.4245, -6.8144) centre (14.4897, -6.7386) ccw
  arc A369 (14.9512, -7.9635) -> (15.0475, -7.9103) centre (14.959, -7.8638) ccw
  arc A370 (13.9179, -7.7971) -> (14.9512, -7.9635) centre (15.4466, -1.5927) ccw
  arc A371 (13.9179, -7.7971) -> (13.807, -7.8448) centre (13.8939, -7.8942) ccw
  arc A372 (15.1594, -7.5596) -> (14.4245, -6.8144) centre (10.2573, -11.6586) ccw
  arc A373 (15.8319, -6.1927) -> (15.8094, -6.0844) centre (15.7391, -6.1556) ccw
  arc A374 (14.9704, -5.2974) -> (15.0069, -5.4124) centre (15.0647, -5.3307) ccw
  arc A375 (15.6405, -6.5062) -> (15.7313, -6.4441) centre (15.6387, -6.4062) ccw
  arc A376 (14.596, -6.4389) -> (15.6405, -6.5062) centre (15.5281, -0.1172) ccw
  arc A377 (14.596, -6.4389) -> (14.4902, -6.4969) centre (14.5814, -6.5378) ccw
  arc A378 (15.8094, -6.0844) -> (15.0069, -5.4124) centre (11.3191, -10.6308) ccw
  arc A379 (16.3489, -4.6598) -> (16.3161, -4.5541) centre (16.2529, -4.6316) ccw
  arc A380 (15.4061, -3.8503) -> (15.4535, -3.9614) centre (15.5032, -3.8746) ccw
  arc A381 (16.1881, -4.99) -> (16.2726, -4.9196) centre (16.1769, -4.8907) ccw
  arc A382 (15.142, -5.0223) -> (16.1881, -4.99) centre (15.4689, 1.3594) ccw
  arc A383 (15.142, -5.0223) -> (15.0421, -5.0901) centre (15.1368, -5.1221) ccw
  arc A384 (16.3161, -4.5541) -> (15.4535, -3.9614) centre (12.2783, -9.5067) ccw
  arc A385 (16.7178, -3.0846) -> (16.6752, -2.9825) centre (16.6196, -3.0657) ccw
  arc A386 (15.7024, -2.3685) -> (15.76, -2.4745) centre (15.8013, -2.3834) ccw
  arc A387 (16.5892, -3.4286) -> (16.6666, -3.3505) centre (16.5685, -3.3308) ccw
  arc A388 (15.5508, -3.5602) -> (16.5892, -3.4286) centre (15.2696, 2.8236) ccw
  arc A389 (15.5508, -3.5602) -> (15.4579, -3.6372) centre (15.5552, -3.6601) ccw
  arc A390 (16.6752, -2.9825) -> (15.76, -2.4745) centre (13.1264, -8.2965) ccw
  arc A391 (16.9353, -1.4815) -> (16.8832, -1.3839) centre (16.8358, -1.472) ccw
  arc A392 (15.8564, -0.8651) -> (15.9239, -0.9652) centre (15.9563, -0.8706) ccw
  arc A393 (16.84, -1.8362) -> (16.9096, -1.7511) centre (16.8101, -1.7408) ccw
  arc A394 (15.8188, -2.0659) -> (16.84, -1.8362) centre (14.9321, 4.2623) ccw
  arc A395 (15.8188, -2.0659) -> (15.7336, -2.1514) centre (15.8327, -2.1649) ccw
  arc A396 (16.8832, -1.3839) -> (15.9239, -0.9652) centre (13.8556, -7.0112) ccw
  arc A397 (15.8669, 0.646) -> (15.8564, 0.8651) centre (0, 0) ccw
  arc A398 (15.7336, 2.1514) -> (15.7024, 2.3685) centre (0, 0) ccw
  arc A399 (15.4579, 3.6372) -> (15.4061, 3.8503) centre (0, 0) ccw
  arc A400 (15.0421, 5.0901) -> (14.9704, 5.2974) centre (0, 0) ccw
  arc A401 (14.4902, 6.4969) -> (14.3991, 6.6964) centre (0, 0) ccw
  arc A402 (13.807, 7.8448) -> (13.6973, 8.0348) centre (0, 0) ccw
  arc A403 (12.9988, 9.1218) -> (12.8715, 9.3004) centre (0, 0) ccw
  arc A404 (12.0728, 10.3161) -> (11.9292, 10.4818) centre (0, 0) ccw
  arc A405 (11.0376, 11.4169) -> (10.8788, 11.5683) centre (0, 0) ccw
  arc A406 (9.9023, 12.4144) -> (9.7299, 12.55) centre (0, 0) ccw
  arc A407 (8.6774, 13.2995) -> (8.4929, 13.4181) centre (0, 0) ccw
  arc A408 (7.3739, 14.0641) -> (7.179, 14.1646) centre (0, 0) ccw
  arc A409 (6.0037, 14.7014) -> (5.8, 14.7829) centre (0, 0) ccw
  arc A410 (4.579, 15.2055) -> (4.3686, 15.2673) centre (0, 0) ccw
  arc A411 (3.1129, 15.5719) -> (2.8976, 15.6134) centre (0, 0) ccw
  arc A412 (1.6186, 15.7973) -> (1.4003, 15.8181) centre (0, 0) ccw
  arc A413 (0.1097, 15.8796) -> (-0.1097, 15.8796) centre (0, 0) ccw
  arc A414 (-1.4003, 15.8181) -> (-1.6186, 15.7973) centre (0, 0) ccw
  arc A415 (-2.8976, 15.6134) -> (-3.1129, 15.5719) centre (0, 0) ccw
  arc A416 (16.9354, 1.4807) -> (16.9096, 1.7511) centre (0, 0) ccw
  arc A417 (16.718, 3.0838) -> (16.6666, 3.3505) centre (0, 0) ccw
  arc A418 (16.3491, 4.659) -> (16.2726, 4.9196) centre (0, 0) ccw
  arc A419 (15.8322, 6.192) -> (15.7313, 6.4441) centre (0, 0) ccw
  arc A420 (15.1719, 7.6689) -> (15.0475, 7.9103) centre (0, 0) ccw
  arc A421 (14.3743, 9.0764) -> (14.2274, 9.3048) centre (0, 0) ccw
  arc A422 (13.4464, 10.4016) -> (13.2785, 10.6151) centre (0, 0) ccw
  arc A423 (12.3968, 11.6327) -> (12.2094, 11.8293) centre (0, 0) ccw
  arc A424 (11.2349, 12.7584) -> (11.0296, 12.9363) centre (0, 0) ccw
  arc A425 (9.9713, 13.7686) -> (9.75, 13.9261) centre (0, 0) ccw
  arc A426 (8.6173, 14.6541) -> (8.3821, 14.7899) centre (0, 0) ccw
  arc A427 (7.1854, 15.4068) -> (6.9383, 15.5197) centre (0, 0) ccw
  arc A428 (5.6883, 16.0201) -> (5.4316, 16.1089) centre (0, 0) ccw
  arc A429 (4.1397, 16.4883) -> (3.8758, 16.5523) centre (0, 0) ccw
  arc A430 (2.5537, 16.8071) -> (2.2849, 16.8458) centre (0, 0) ccw
  arc A431 (0.9445, 16.9737) -> (0.6732, 16.9867) centre (0, 0) ccw
  arc A432 (-0.6732, 16.9867) -> (-0.9445, 16.9737) centre (0, 0) ccw
  arc A433 (-2.2849, 16.8458) -> (-2.5537, 16.8071) centre (0, 0) ccw
  arc A434 (16.9995, -0.1358) -> (16.9995, 0.1358) centre (0, 0) ccw
  arc A435 (15.8564, -0.8651) -> (15.8669, -0.646) centre (0, 0) ccw
  arc A436 (-4.3686, 15.2673) -> (-4.579, 15.2055) centre (0, 0) ccw
  arc A437 (-5.8, 14.7829) -> (-6.0037, 14.7014) centre (0, 0) ccw
  arc A438 (-7.179, 14.1646) -> (-7.3739, 14.0641) centre (0, 0) ccw
  arc A439 (-8.4929, 13.4181) -> (-8.6774, 13.2995) centre (0, 0) ccw
  arc A440 (-9.7299, 12.55) -> (-9.9023, 12.4144) centre (0, 0) ccw
  arc A441 (-10.8788, 11.5683) -> (-11.0376, 11.4169) centre (0, 0) ccw
  arc A442 (-11.9292, 10.4818) -> (-12.0728, 10.3161) centre (0, 0) ccw
  arc A443 (-12.8715, 9.3004) -> (-12.9988, 9.1218) centre (0, 0) ccw
  arc A444 (-13.6973, 8.0348) -> (-13.807, 7.8448) centre (0, 0) ccw
  arc A445 (-14.3991, 6.6964) -> (-14.4902, 6.4969) centre (0, 0) ccw
  arc A446 (-14.9704, 5.2974) -> (-15.0421, 5.0901) centre (0, 0) ccw
  arc A447 (-15.4061, 3.8503) -> (-15.4579, 3.6372) centre (0, 0) ccw
  arc A448 (-15.7024, 2.3685) -> (-15.7336, 2.1514) centre (0, 0) ccw
  arc A449 (-15.8564, 0.8651) -> (-15.8669, 0.646) centre (0, 0) ccw
  arc A450 (-15.8669, -0.646) -> (-15.8564, -0.8651) centre (0, 0) ccw
  arc A451 (-15.7336, -2.1514) -> (-15.7024, -2.3685) centre (0, 0) ccw
  arc A452 (-15.4579, -3.6372) -> (-15.4061, -3.8503) centre (0, 0) ccw
  arc A453 (-15.0421, -5.0901) -> (-14.9704, -5.2974) centre (0, 0) ccw
  arc A454 (-14.4902, -6.4969) -> (-14.3991, -6.6964) centre (0, 0) ccw
  arc A455 (-13.807, -7.8448) -> (-13.6973, -8.0348) centre (0, 0) ccw
  arc A456 (-12.9988, -9.1218) -> (-12.8715, -9.3004) centre (0, 0) ccw
  arc A457 (-12.0728, -10.3161) -> (-11.9292, -10.4818) centre (0, 0) ccw
  arc A458 (-11.0376, -11.4169) -> (-10.8788, -11.5683) centre (0, 0) ccw
  arc A459 (-9.9023, -12.4144) -> (-9.7299, -12.55) centre (0, 0) ccw
  arc A460 (-3.8758, 16.5523) -> (-4.1397, 16.4883) centre (0, 0) ccw
  arc A461 (-5.4316, 16.1089) -> (-5.6883, 16.0201) centre (0, 0) ccw
  arc A462 (-6.9383, 15.5197) -> (-7.1854, 15.4068) centre (0, 0) ccw
  arc A463 (-8.3821, 14.7899) -> (-8.6173, 14.6541) centre (0, 0) ccw
  arc A464 (-9.75, 13.9261) -> (-9.9713, 13.7686) centre (0, 0) ccw
  arc A465 (-11.0296, 12.9363) -> (-11.2349, 12.7584) centre (0, 0) ccw
  arc A466 (-12.2094, 11.8293) -> (-12.3968, 11.6327) centre (0, 0) ccw
  arc A467 (-13.2785, 10.6151) -> (-13.4464, 10.4016) centre (0, 0) ccw
  arc A468 (-14.2274, 9.3048) -> (-14.3743, 9.0764) centre (0, 0) ccw
  arc A469 (-15.0475, 7.9103) -> (-15.1719, 7.6689) centre (0, 0) ccw
  arc A470 (-15.7313, 6.4441) -> (-15.8322, 6.192) centre (0, 0) ccw
  arc A471 (-16.2726, 4.9196) -> (-16.3491, 4.659) centre (0, 0) ccw
  arc A472 (-16.6666, 3.3505) -> (-16.718, 3.0838) centre (0, 0) ccw
  arc A473 (-16.9096, 1.7511) -> (-16.9354, 1.4807) centre (0, 0) ccw
  arc A474 (-16.9995, 0.1358) -> (-16.9995, -0.1358) centre (0, 0) ccw
  arc A475 (-16.9354, -1.4807) -> (-16.9096, -1.7511) centre (0, 0) ccw
  arc A476 (-16.718, -3.0838) -> (-16.6666, -3.3505) centre (0, 0) ccw
  arc A477 (-16.3491, -4.659) -> (-16.2726, -4.9196) centre (0, 0) ccw
  arc A478 (-15.8322, -6.192) -> (-15.7313, -6.4441) centre (0, 0) ccw
  arc A479 (-15.1719, -7.6689) -> (-15.0475, -7.9103) centre (0, 0) ccw
  arc A480 (-14.3743, -9.0764) -> (-14.2274, -9.3048) centre (0, 0) ccw
  arc A481 (-13.4464, -10.4016) -> (-13.2785, -10.6151) centre (0, 0) ccw
  arc A482 (-12.3968, -11.6327) -> (-12.2094, -11.8293) centre (0, 0) ccw
  arc A483 (-11.2349, -12.7584) -> (-11.0296, -12.9363) centre (0, 0) ccw
  arc A484 (16.9096, -1.7511) -> (16.9354, -1.4807) centre (0, 0) ccw
  arc A485 (16.6666, -3.3505) -> (16.718, -3.0838) centre (0, 0) ccw
  arc A486 (16.2726, -4.9196) -> (16.3491, -4.659) centre (0, 0) ccw
  arc A487 (15.7313, -6.4441) -> (15.8322, -6.192) centre (0, 0) ccw
  arc A488 (15.0475, -7.9103) -> (15.1719, -7.6689) centre (0, 0) ccw
  arc A489 (14.2274, -9.3048) -> (14.3743, -9.0764) centre (0, 0) ccw
  arc A490 (13.2785, -10.6151) -> (13.4464, -10.4016) centre (0, 0) ccw
  arc A491 (12.2094, -11.8293) -> (12.3968, -11.6327) centre (0, 0) ccw
  arc A492 (11.0296, -12.9363) -> (11.2349, -12.7584) centre (0, 0) ccw
  arc A493 (9.75, -13.9261) -> (9.9713, -13.7686) centre (0, 0) ccw
  arc A494 (8.3821, -14.7899) -> (8.6173, -14.6541) centre (0, 0) ccw
  arc A495 (6.9383, -15.5197) -> (7.1854, -15.4068) centre (0, 0) ccw
  arc A496 (5.4316, -16.1089) -> (5.6883, -16.0201) centre (0, 0) ccw
  arc A497 (3.8758, -16.5523) -> (4.1397, -16.4883) centre (0, 0) ccw
  arc A498 (2.2849, -16.8458) -> (2.5537, -16.8071) centre (0, 0) ccw
  arc A499 (0.6732, -16.9867) -> (0.9445, -16.9737) centre (0, 0) ccw
  arc A500 (-0.9445, -16.9737) -> (-0.6732, -16.9867) centre (0, 0) ccw
  arc A501 (-2.5537, -16.8071) -> (-2.2849, -16.8458) centre (0, 0) ccw
  arc A502 (-4.1397, -16.4883) -> (-3.8758, -16.5523) centre (0, 0) ccw
  arc A503 (-5.6883, -16.0201) -> (-5.4316, -16.1089) centre (0, 0) ccw
  arc A504 (-7.1854, -15.4068) -> (-6.9383, -15.5197) centre (0, 0) ccw
  arc A505 (-9.9713, -13.7686) -> (-9.75, -13.9261) centre (0, 0) ccw
  arc A506 (-8.6173, -14.6541) -> (-8.3821, -14.7899) centre (0, 0) ccw
  arc A507 (15.7024, -2.3685) -> (15.7336, -2.1514) centre (0, 0) ccw
  arc A508 (15.4061, -3.8503) -> (15.4579, -3.6372) centre (0, 0) ccw
  arc A509 (14.9704, -5.2974) -> (15.0421, -5.0901) centre (0, 0) ccw
  arc A510 (14.3991, -6.6964) -> (14.4902, -6.4969) centre (0, 0) ccw
  arc A511 (13.6973, -8.0348) -> (13.807, -7.8448) centre (0, 0) ccw
  arc A512 (12.8715, -9.3004) -> (12.9988, -9.1218) centre (0, 0) ccw
  arc A513 (11.9292, -10.4818) -> (12.0728, -10.3161) centre (0, 0) ccw
  arc A514 (10.8788, -11.5683) -> (11.0376, -11.4169) centre (0, 0) ccw
  arc A515 (9.7299, -12.55) -> (9.9023, -12.4144) centre (0, 0) ccw
  arc A516 (8.4929, -13.4181) -> (8.6774, -13.2995) centre (0, 0) ccw
  arc A517 (7.179, -14.1646) -> (7.3739, -14.0641) centre (0, 0) ccw
  arc A518 (5.8, -14.7829) -> (6.0037, -14.7014) centre (0, 0) ccw
  arc A519 (4.3686, -15.2673) -> (4.579, -15.2055) centre (0, 0) ccw
  arc A520 (2.8976, -15.6134) -> (3.1129, -15.5719) centre (0, 0) ccw
  arc A521 (1.4003, -15.8181) -> (1.6186, -15.7973) centre (0, 0) ccw
  arc A522 (-0.1097, -15.8796) -> (0.1097, -15.8796) centre (0, 0) ccw
  arc A523 (-1.6186, -15.7973) -> (-1.4003, -15.8181) centre (0, 0) ccw
  arc A524 (-3.1129, -15.5719) -> (-2.8976, -15.6134) centre (0, 0) ccw
  arc A525 (-4.579, -15.2055) -> (-4.3686, -15.2673) centre (0, 0) ccw
  arc A526 (-6.0037, -14.7014) -> (-5.8, -14.7829) centre (0, 0) ccw
  arc A527 (-8.6774, -13.2995) -> (-8.4929, -13.4181) centre (0, 0) ccw
  arc A528 (-7.3739, -14.0641) -> (-7.179, -14.1646) centre (0, 0) ccw
  point P0 (16.9988, 0.2013)
  point P1 (15.8698, 0.57)
  point P2 (16.9904, 0.57)
  point P3 (16.9988, -0.2013)
  point P4 (15.8698, -0.57)
  point P5 (16.941, 1.4154)
  point P6 (15.8521, 0.9411)
  point P7 (16.9027, 1.8162)
  point P8 (15.7437, 2.0759)
  point P9 (16.8593, 2.1825)
  point P10 (16.7297, 3.0194)
  point P11 (15.6909, 2.4437)
  point P12 (16.6535, 3.4147)
  point P13 (15.4751, 3.5631)
  point P14 (16.5755, 3.7752)
  point P15 (16.367, 4.596)
  point P16 (15.3875, 3.9241)
  point P17 (16.2535, 4.9823)
  point P18 (15.0663, 5.0179)
  point P19 (16.1416, 5.3337)
  point P20 (15.856, 6.1309)
  point P21 (14.9448, 5.369)
  point P22 (15.7063, 6.5047)
  point P23 (14.5211, 6.4274)
  point P24 (15.5615, 6.8439)
  point P25 (15.2014, 7.6104)
  point P26 (14.3668, 6.7653)
  point P27 (15.0169, 7.9682)
  point P28 (13.8444, 7.7786)
  point P29 (14.8405, 8.2921)
  point P30 (14.4091, 9.0209)
  point P31 (13.6587, 8.1003)
  point P32 (14.1915, 9.3596)
  point P33 (13.0423, 9.0594)
  point P34 (13.9851, 9.6652)
  point P35 (13.4864, 10.3497)
  point P36 (12.8268, 9.362)
  point P37 (13.2375, 10.6662)
  point P38 (12.1221, 10.2581)
  point P39 (13.003, 10.9508)
  point P40 (12.4415, 11.5848)
  point P41 (11.8788, 10.5389)
  point P42 (12.1637, 11.8762)
  point P43 (11.0921, 11.3639)
  point P44 (11.9032, 12.1373)
  point P45 (11.284, 12.715)
  point P46 (10.8233, 11.6203)
  point P47 (10.9797, 12.9787)
  point P48 (9.9617, 12.3668)
  point P49 (10.6956, 13.2138)
  point P50 (10.0243, 13.73)
  point P51 (9.6697, 12.5965)
  point P52 (9.6963, 13.9636)
  point P53 (8.7411, 13.2578)
  point P54 (9.3911, 14.1706)
  point P55 (8.6737, 14.6207)
  point P56 (8.4285, 13.4586)
  point P57 (8.3251, 14.8221)
  point P58 (7.4412, 14.0286)
  point P59 (8.0016, 14.9992)
  point P60 (7.2447, 15.379)
  point P61 (7.111, 14.1989)
  point P62 (6.8784, 15.5463)
  point P63 (6.074, 14.6724)
  point P64 (6.5396, 15.6918)
  point P65 (5.75, 15.998)
  point P66 (5.7291, 14.8105)
  point P67 (5.3695, 16.1297)
  point P68 (4.6518, 15.1834)
  point P69 (5.0184, 16.2424)
  point P70 (4.2033, 16.4722)
  point P71 (4.2954, 15.288)
  point P72 (3.812, 16.5671)
  point P73 (3.1875, 15.5568)
  point P74 (3.4517, 16.6459)
  point P75 (2.6184, 16.7971)
  point P76 (2.8227, 15.6271)
  point P77 (2.2199, 16.8544)
  point P78 (1.6943, 15.7894)
  point P79 (1.8538, 16.8986)
  point P80 (1.0099, 16.97)
  point P81 (1.3245, 15.8247)
  point P82 (0.6078, 16.9891)
  point P83 (0.1858, 15.8789)
  point P84 (0.2391, 16.9983)
  point P85 (-0.6078, 16.9891)
  point P86 (-0.1858, 15.8789)
  point P87 (-1.0099, 16.97)
  point P88 (-1.3245, 15.8247)
  point P89 (-1.3778, 16.9441)
  point P90 (-2.2199, 16.8544)
  point P91 (-1.6943, 15.7894)
  point P92 (-2.6184, 16.7971)
  point P93 (-2.8227, 15.6271)
  point P94 (-2.9822, 16.7364)
  point P95 (-3.812, 16.5671)
  point P96 (-3.1875, 15.5568)
  point P97 (-4.2033, 16.4722)
  point P98 (-4.2954, 15.288)
  point P99 (-4.5596, 16.3771)
  point P100 (-5.3695, 16.1297)
  point P101 (-4.6518, 15.1834)
  point P102 (-5.75, 15.998)
  point P103 (-5.7291, 14.8105)
  point P104 (-6.0957, 15.8696)
  point P105 (-6.8784, 15.5463)
  point P106 (-6.074, 14.6724)
  point P107 (-7.2447, 15.379)
  point P108 (-7.111, 14.1989)
  point P109 (-7.5766, 15.2183)
  point P110 (-8.3251, 14.8221)
  point P111 (-7.4412, 14.0286)
  point P112 (-8.6737, 14.6207)
  point P113 (-8.4285, 13.4586)
  point P114 (-8.9889, 14.4292)
  point P115 (-9.6963, 13.9636)
  point P116 (-8.7411, 13.2578)
  point P117 (-10.0243, 13.73)
  point P118 (-9.6697, 12.5965)
  point P119 (-10.3197, 13.5094)
  point P120 (-10.9797, 12.9787)
  point P121 (-9.9617, 12.3668)
  point P122 (-11.284, 12.715)
  point P123 (-10.8233, 11.6203)
  point P124 (-11.5572, 12.4672)
  point P125 (-12.1637, 11.8762)
  point P126 (-11.0921, 11.3639)
  point P127 (-12.4415, 11.5848)
  point P128 (-11.8788, 10.5389)
  point P129 (-12.6899, 11.3122)
  point P130 (-13.2375, 10.6662)
  point P131 (-12.1221, 10.2581)
  point P132 (-13.4864, 10.3497)
  point P133 (-12.8268, 9.362)
  point P134 (-13.7077, 10.0547)
  point P135 (-14.1915, 9.3596)
  point P136 (-13.0423, 9.0594)
  point P137 (-14.4091, 9.0209)
  point P138 (-13.6587, 8.1003)
  point P139 (-14.6014, 8.7062)
  point P140 (-15.0169, 7.9682)
  point P141 (-13.8444, 7.7786)
  point P142 (-15.2014, 7.6104)
  point P143 (-14.3668, 6.7653)
  point P144 (-15.3629, 7.2788)
  point P145 (-15.7063, 6.5047)
  point P146 (-14.5211, 6.4274)
  point P147 (-15.856, 6.1309)
  point P148 (-14.9448, 5.369)
  point P149 (-15.9852, 5.7855)
  point P150 (-16.2535, 4.9823)
  point P151 (-15.0663, 5.0179)
  point P152 (-16.367, 4.596)
  point P153 (-15.3875, 3.9241)
  point P154 (-16.4628, 4.2398)
  point P155 (-16.6535, 3.4147)
  point P156 (-15.4751, 3.5631)
  point P157 (-16.7297, 3.0194)
  point P158 (-15.6909, 2.4437)
  point P159 (-16.7913, 2.6558)
  point P160 (-16.9027, 1.8162)
  point P161 (-15.7437, 2.0759)
  point P162 (-16.941, 1.4154)
  point P163 (-15.8521, 0.9411)
  point P164 (-16.9677, 1.0476)
  point P165 (-16.9988, 0.2013)
  point P166 (-15.8698, 0.57)
  point P167 (-16.9988, -0.2013)
  point P168 (-15.8698, -0.57)
  point P169 (-16.9904, -0.57)
  point P170 (-16.941, -1.4154)
  point P171 (-15.8521, -0.9411)
  point P172 (-16.9027, -1.8162)
  point P173 (-15.7437, -2.0759)
  point P174 (-16.8593, -2.1825)
  point P175 (-16.7297, -3.0194)
  point P176 (-15.6909, -2.4437)
  point P177 (-16.6535, -3.4147)
  point P178 (-15.4751, -3.5631)
  point P179 (-16.5755, -3.7752)
  point P180 (-16.367, -4.596)
  point P181 (-15.3875, -3.9241)
  point P182 (-16.2535, -4.9823)
  point P183 (-15.0663, -5.0179)
  point P184 (-16.1416, -5.3337)
  point P185 (-15.856, -6.1309)
  point P186 (-14.9448, -5.369)
  point P187 (-15.7063, -6.5047)
  point P188 (-14.5211, -6.4274)
  point P189 (-15.5615, -6.8439)
  point P190 (-15.2014, -7.6104)
  point P191 (-14.3668, -6.7653)
  point P192 (-15.0169, -7.9682)
  point P193 (-13.8444, -7.7786)
  point P194 (-14.8405, -8.2921)
  point P195 (-14.4091, -9.0209)
  point P196 (-13.6587, -8.1003)
  point P197 (-14.1915, -9.3596)
  point P198 (-13.0423, -9.0594)
  point P199 (-13.9851, -9.6652)
  dimension "d0" = 15
  dimension "d3" = 0.135
  dimension "d4" = 0.57
  dimension "d5" = 0.2
  dimension "d6" = 0.2
  dimension "d7" = 6.39
  dimension "d10" = 360
  constraints: 858 point on circle, 397 centre point, 6 end point, 5 symmetric about line, 4 point on line, 3 horizontal, 2 horizontal alignment, 2 tangent, 2 vertical alignment, 2115 other
  measures "d0" diameter of A0
  measures "d3" distance between parallel lines of L2 L0
  measures "d4" distance between parallel lines of L1 L0
  measures "d5" diameter of A2
  measures "d6" diameter of A3
  measures "d7" radius of A1
extrude "Extrusion1" add sketch "Sketch1" along normal blind 7
sketch "Sketch2" plane through (7, 0, 0) normal (1, 0, 0) x (0, 0, -1)
  circle A0 centre (0, 0) radius 10
  circle A1 centre (0, 0) radius 7.5 projected
  dimension "d14" = 20
  constraints: 1 centre point, 1 coincident
  measures "d14" diameter of A0
extrude "Extrusion2" add sketch "Sketch2" along normal blind 2
chamfer "Chamfer1" distance 0.5 angle 45 1 edges at (9, 0, 10)
fillet "Fillet1" radius 0.1 5 edges at (8.5, 0, 10) (9, 0, 9.5) (9, 0, 7.5) (7, 0, 10) (0, -7.5, 0)